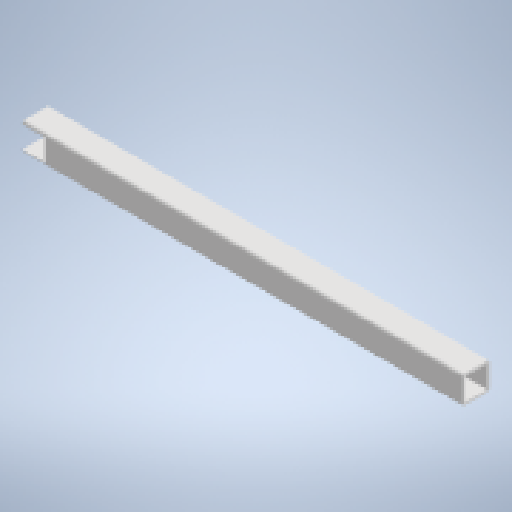
# Autodesk Inventor part: rockerpivotarm
Saved by Autodesk Inventor 2025.2 (Build 292293000, 293)
## iProperties
Created: 2026-03-21
Part Number: rockerpivotarm
Material: Generic
Document SubType Name: Modeling
Designer: hp
Density: 1 g/cm^3
Appearance: Default
Author: hp
Autodesk Inventor part; units mm, degrees
ref_plane "YZ Plane" through (0, 0, 0) normal (1, 0, 0) x (0, 1, 0)
ref_plane "XZ Plane" through (0, 0, 0) normal (0, 1, 0) x (-1, 0, 0)
ref_plane "XY Plane" through (0, 0, 0) normal (0, 0, 1) x (1, 0, 0)
sketch "Sketch1" plane through (0, 0, 0) normal (1, 0, 0) x (0, 1, 0)
  line L0 (2, 0) -> (18, 0)
  line L1 (20, -2) -> (20, -18)
  line L2 (18, -20) -> (2, -20)
  line L3 (0, -18) -> (0, -2)
  line L4 (18, -18) -> (18, -2)
  line L5 (18, -2) -> (2, -2)
  line L6 (2, -2) -> (2, -18)
  line L7 (2, -18) -> (18, -18)
  arc A0 (20, -2) -> (18, 0) centre (18, -2) ccw
  arc A1 (18, -20) -> (20, -18) centre (18, -18) ccw
  arc A2 (0, -18) -> (2, -20) centre (2, -18) ccw
  arc A3 (2, 0) -> (0, -2) centre (2, -2) ccw
  point P0 (0, 0)
  point P1 (20, -20)
  point P2 (20, 0)
  point P3 (0, -20)
  dimension "d0" = 20
  dimension "d1" = 20
  dimension "d2" = 2
  dimension "d5" = 2
  constraints: 16 end point, 8 point on circle, 8 point on line, 8 tangent, 4 centre point, 4 parallel, 3 equal radius, 2 perpendicular, 1 horizontal, 3 other
  measures "d0" distance of point (20, -20) point (0, -20)
  measures "d1" distance of point (20, 0) point (20, -20)
  measures "d2" distance between parallel lines of L1 L4
  measures "d5" radius of A0
extrude "Extrusion1" add sketch "Sketch1" along normal blind 319
sketch "Sketch2" plane through (0, 0, -18) normal (0, -1, 0) x (1, 0, 0)
  line L0 (0, 16) -> (0, 0) projected
  line L1 (0, 0) -> (319, 0) projected
  point P0 (0, 18)
  point P1 (16, 8)
  dimension "d6" = 16
  dimension "d7" = 8
  measures "d6" distance from line of point (16, 8) L0
  measures "d7" distance from line of point (16, 8) L1
hole "Hole1" at (16, 0, -10) direction (0, 1, 0) diameter 2.45 depth 2 tip angle 118
sketch "Sketch3" plane through (0, 2, 0) normal (0, 0, 1) x (1, 0, 0)
  line L0 (0, 0) -> (319, 0) projected
  line L1 (0, 0) -> (16, 0)
  line L2 (16, 0) -> (16, 16)
  line L3 (16, 16) -> (0, 16)
  line L4 (0, 16) -> (0, 0)
  point P0 (0, -2)
  dimension "d15" = 16
  dimension "d16" = 16
  constraints: 8 end point, 2 parallel, 1 horizontal, 1 perpendicular
  measures "d15" distance of L3.end L2.end
  measures "d16" distance of L2.end L1.end
extrude "Extrusion2" cut sketch "Sketch3" against normal up to surface (2 mm away)
body "Solid1"
